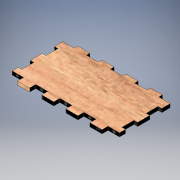
# Autodesk Inventor part: LeftRigthPlate
Saved by Autodesk Inventor 2019.4 (Build 234330000, 330)
## iProperties
Created: 2020-06-30
Part Number: LeftRigthPlate
Material: Wood (Birch)
Document SubType Name: Modeling
Designer: wimva
Density: 0.55 g/cm^3
Appearance: Birch - Natural Polished
Author: wimva
Autodesk Inventor part; units mm, degrees
ref_plane "YZ Plane" through (0, 0, 0) normal (1, 0, 0) x (0, 1, 0)
ref_plane "XZ Plane" through (0, 0, 0) normal (0, 1, 0) x (-1, 0, 0)
ref_plane "XY Plane" through (0, 0, 0) normal (0, 0, 1) x (1, 0, 0)
sketch "Sketch1" plane through (0, 0, 0) normal (0, 1, 0) x (1, 0, 0)
  line L0 (44.5, -25) -> (-44.5, -25)
  line L1 (-44.5, -25) -> (-44.5, 25)
  line L2 (-44.5, 25) -> (44.5, 25)
  line L3 (44.5, 25) -> (44.5, -25)
  line L4 (44.5, -25) -> (-44.5, 25) construction
  line L5 (-44.5, -25) -> (44.5, 25) construction
  point P0 (0, 0)
  dimension "d0" = 89
  dimension "d1" = 50
  constraints: 12 end point, 2 midpoint, 2 parallel, 1 horizontal, 1 perpendicular
  measures "d0" distance of L1.end L2.end
  measures "d1" distance of L2.end L0.start
extrude "Extrusion1" add sketch "Sketch1" along normal blind 3
sketch "Sketch2" plane through (0, 3, 0) normal (0, 1, 0) x (1, 0, 0)
  line L0 (44.5, 25) -> (-44.5, 25) construction
  line L1 (-5, 25) -> (5, 25)
  line L2 (5, 25) -> (5, 22)
  line L3 (5, 22) -> (-5, 22)
  line L4 (-5, 22) -> (-5, 25)
  line L5 (0, 35) -> (0, -35) construction
  point P0 (0, 0)
  dimension "d4" = 10
  dimension "d5" = 3
  constraints: 8 end point, 2 parallel, 1 horizontal, 1 perpendicular, 1 point on line, 1 other
  measures "d4" distance of L2.end L3.end
  measures "d5" distance of L1.end L2.end
extrude "Extrusion2" cut sketch "Sketch2" against normal through all
pattern_linear "Rectangular Pattern1" count 3 spacing 20 along (-1, 0, 0) count 2 spacing 40 along (1, 0, 0) of "Extrusion2"
sketch "Sketch3" plane through (0, 3, 0) normal (0, 1, 0) x (1, 0, 0)
  line L0 (-44.5, -15) -> (-41.5, -15)
  line L1 (-41.5, -15) -> (-41.5, -5)
  line L2 (-41.5, -5) -> (-44.5, -5)
  line L3 (-44.5, -5) -> (-44.5, -15)
  line L4 (-44.5, 25) -> (-44.5, -25) construction
  line L5 (62.3, 0) -> (-62.3, 0) construction
  point P0 (0, 0)
  dimension "d15" = 3
  dimension "d16" = 10
  dimension "d17" = 5
  constraints: 8 end point, 2 parallel, 1 collinear, 1 horizontal, 1 perpendicular
  measures "d15" distance of L2.end L1.end
  measures "d16" distance of L1.end L0.end
  measures "d17" distance between parallel lines of L5 L2
extrude "Extrusion3" cut sketch "Sketch3" against normal blind 3
pattern_linear "Rectangular Pattern2" count 2 spacing 20 along (0, 0, -1) of "Extrusion3"
mirror "Mirror2" about plane through (0, 0, 0) normal (1, 0, 0) of "Extrusion3", "Rectangular Pattern2"
sketch "Sketch4" plane through (0, 3, 0) normal (0, 1, 0) x (1, 0, 0)
  line L0 (-44.5, -25) -> (44.5, -25) construction
  line L1 (-5, -25) -> (5, -25)
  line L2 (5, -25) -> (5, -20)
  line L3 (5, -20) -> (-5, -20)
  line L4 (-5, -20) -> (-5, -25)
  line L5 (0, 35) -> (0, -35) construction
  point P0 (0, 0)
  dimension "d23" = 10
  dimension "d24" = 5
  constraints: 8 end point, 2 parallel, 1 horizontal, 1 perpendicular, 1 point on line, 1 other
  measures "d23" distance of L3.end L2.end
  measures "d24" distance of L1.end L2.end
extrude "Extrusion4" cut sketch "Sketch4" against normal through all
pattern_linear "Rectangular Pattern3" count 3 spacing 20 along (-1, 0, 0) count 2 spacing 40 along (1, 0, 0) of "Extrusion4"
equation "\"d0\" = Module_Height"
equation "\"d1\" = Module_Depth"
equation "\"d2\" = Module_Case_Thickness"
equation "\"d4\" = Module_Case_SlotWidth"
equation "\"d5\" = Module_Case_SlotDepth"
equation "\"d7\" = Module_Case_Thickness"
equation "\"d11\" = 2 * Module_Case_SlotWidth"
equation "\"d14\" = 4 * Module_Case_SlotWidth"
equation "\"d15\" = Module_Case_SlotDepth"
equation "\"d16\" = Module_Case_SlotWidth"
equation "\"d17\" = 0.5 * Module_Case_SlotWidth"
equation "\"d18\" = Module_Case_Thickness"
equation "\"d22\" = 2 * Module_Case_SlotWidth"
equation "\"d23\" = Module_Case_SlotWidth"
equation "\"d24\" = Module_Case_BottomSlotDepth"
equation "\"d30\" = 2 * Module_Case_SlotWidth"
equation "\"d33\" = 4 * Module_Case_SlotWidth"
equation "\"RackWidth\" = 482.6"
equation "\"U\" = 44.5"
equation "\"Module_Connector_Width\" = 6"
equation "\"Module_Case_SlotWidth\" = 10"
equation "\"Module_Case_SlotDepth\" = 3"
equation "\"Module_Depth\" = 50"
equation "\"Module_Back_Thickness\" = 5"
equation "\"Module_Connector_Depth\" = 4"
equation "\"Module_Height\" = 89"
equation "\"Module_Width\" = 96.52"
equation "\"Module_Case_Thickness\" = 3"
equation "\"Module_StatusIndicatorDiameter\" = 5"
equation "\"Module_Case_BottomSlotDepth\" = 5"
body "Solid1"
